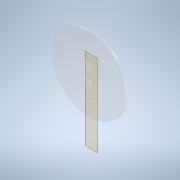
# Autodesk Inventor part: szklo
Saved by Autodesk Inventor 2021 (Build 250183000, 183)
## iProperties
Created: 2021-11-16
Part Number: szklo
Material: Akrylowy, przezroczysty
Document SubType Name: Modeling
Designer: wojwo
Density: 1.19 g/cm^3
Appearance: Przezroczyste — przejrzyste
Author: wojwo
Autodesk Inventor part; units mm, degrees
ref_plane "YZ Plane" through (0, 0, 0) normal (1, 0, 0) x (0, 1, 0)
ref_plane "XZ Plane" through (0, 0, 0) normal (0, 1, 0) x (-1, 0, 0)
ref_plane "XY Plane" through (0, 0, 0) normal (0, 0, 1) x (1, 0, 0)
ref_plane "Płaszczyzna konstrukcyjna1" through (0, 0, 0) normal (0, 0, 1) x (1, 0, 0)
sketch "Szkic1" plane through (0, 0, 0) normal (0, 0, 1) x (1, 0, 0)
  circle A0 centre (0, 20) radius 2.5 projected
  circle A1 centre (0, 35) radius 2.5 projected
  circle A2 centre (0, 27.5) radius 40
  point P0 (0, 0)
  dimension "d0" = 7.5
  dimension "d1" = 7.5
  dimension "d2" = 80
  constraints: 1 centre point, 1 coincident
  measures "d0" distance of A0.centre point (0, 27.5)
  measures "d1" distance of A1.centre point (0, 27.5)
  measures "d2" diameter of A2
extrude "Wyciągnięcie proste1" add sketch "Szkic1" along normal blind 3
chamfer "Faza1" distance 0.4 angle 45 2 edges at (-40, 27.5, 3) (-40, 27.5, 0)
chamfer "Faza3" distance 2 angle 45 2 edges at (-2.5, 20, 3) (-2.5, 35, 3)
sketch "Szkic2" plane through (0, 27.5, 0) normal (0, 0, -1) x (-1, 0, 0)
  point P0 (0, -27.5)
sketch "Szkic3" plane through (0, 27.5, 0) normal (0, 0, -1) x (-1, 0, 0)
  point P0 (0, -27.5)
